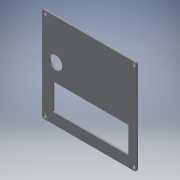
# Autodesk Inventor part: covor
Saved by Autodesk Inventor 2019 (Build 230136000, 136)
## iProperties
Created: 2021-10-12
Part Number: covor
Material: Generic
Document SubType Name: Modeling
Designer: Pulag
Density: 1 g/cm^3
Appearance: Default
Author: Pulag
Autodesk Inventor part; units mm, degrees
ref_plane "YZ Plane" through (0, 0, 0) normal (1, 0, 0) x (0, 1, 0)
ref_plane "XZ Plane" through (0, 0, 0) normal (0, 1, 0) x (-1, 0, 0)
ref_plane "XY Plane" through (0, 0, 0) normal (0, 0, 1) x (1, 0, 0)
sketch "Sketch1" plane through (0, 0, 0) normal (0, 0, 1) x (1, 0, 0)
  arc A0 (-45, -43.5) -> (-43.5, -45) centre (-43.5, -43.5) ccw projected
  line L0 (-43.5, -45) -> (43.5, -45) projected
  arc A1 (43.5, -45) -> (45, -43.5) centre (43.5, -43.5) ccw projected
  line L1 (45, -43.5) -> (45, 4.25) projected
  line L2 (45, 4.25) -> (42.25, 4.25) projected
  line L3 (42.25, 4.25) -> (42.25, -40.75) projected
  arc A2 (40.75, -42.25) -> (42.25, -40.75) centre (42.25, -42.25) ccw projected
  line L4 (40.75, -42.25) -> (-40.75, -42.25) projected
  arc A3 (-42.25, -40.75) -> (-40.75, -42.25) centre (-42.25, -42.25) ccw projected
  line L5 (-42.25, -40.75) -> (-42.25, 40.75) projected
  arc A4 (-40.75, 42.25) -> (-42.25, 40.75) centre (-42.25, 42.25) ccw projected
  line L6 (-40.75, 42.25) -> (-5, 42.25) projected
  line L7 (-5, 42.25) -> (-5, 45) projected
  line L8 (-5, 45) -> (-43.5, 45) projected
  arc A5 (-43.5, 45) -> (-45, 43.5) centre (-43.5, 43.5) ccw projected
  line L9 (-45, 43.5) -> (-45, -43.5) projected
  line L10 (-45, 45) -> (45, 45)
  line L11 (45, 45) -> (45, -45)
  line L12 (45, -45) -> (-45, -45)
  line L13 (-45, -45) -> (-45, 45)
  line L14 (-45, 45) -> (45, -45) construction
  line L15 (45, 45) -> (-45, -45) construction
  line L16 (37.25, -9.75) -> (-34.75, -9.75)
  line L17 (-34.75, -9.75) -> (-34.75, -34.75)
  line L18 (-34.75, -34.75) -> (37.25, -34.75)
  line L19 (37.25, -34.75) -> (37.25, -9.75)
  circle A6 centre (-32, 7) radius 6.25
  point P0 (0, 0)
  dimension "d9" = 1.5
  dimension "d0" = 90
  dimension "d1" = 90
  dimension "d2" = 72
  dimension "d3" = 25
  dimension "d4" = 7.5
  dimension "d5" = 5
  dimension "d6" = 12.5
  dimension "d19" = 38
  dimension "d20" = 13
  constraints: 20 end point, 4 parallel, 2 horizontal, 2 midpoint, 2 perpendicular, 1 centre point
  measures "d0" distance of L10.end L11.end
  measures "d1" distance between parallel lines of L9 L11
  measures "d2" distance of L18.end L17.end
  measures "d3" distance of L17.end L16.end
  measures "d4" distance between parallel lines of L4 L18
  measures "d5" distance between parallel lines of L3 L19
  measures "d6" diameter of A6
  measures "d19" distance from line of L8 A6.centre
  measures "d20" distance from line of L9 A6.centre
extrude "Extrusion1" add sketch "Sketch1" along normal blind 1.5
fillet "Fillet1" radius 2 4 edges at (45, -45, 0.75) (-45, -45, 0.75) (-45, 45, 0.75) (45, 45, 0.75)
sketch "Sketch2" plane through (0, 0, 1.5) normal (0, 0, 1) x (1, 0, 0)
  arc A0 (40.75, -42.25) -> (42.25, -40.75) centre (42.25, -42.25) ccw projected
  arc A1 (-42.25, -40.75) -> (-40.75, -42.25) centre (-42.25, -42.25) ccw projected
  arc A2 (-40.75, 42.25) -> (-42.25, 40.75) centre (-42.25, 42.25) ccw projected
  arc A3 (42.25, 40.75) -> (40.75, 42.25) centre (42.25, 42.25) ccw projected
  circle A4 centre (42.25, 42.25) radius 1.65
  circle A5 centre (-42.25, 42.25) radius 1.65
  circle A6 centre (-42.25, -42.25) radius 1.65
  circle A7 centre (42.25, -42.25) radius 1.65
  point P0 (0, 0)
  dimension "d12" = 3.3
  dimension "d13" = 3.3
  dimension "d14" = 3.3
  dimension "d15" = 3.3
  constraints: 4 centre point, 4 coincident
  measures "d12" diameter of A4
  measures "d13" diameter of A5
  measures "d14" diameter of A6
  measures "d15" diameter of A7
extrude "Extrusion2" cut sketch "Sketch2" against normal blind 3
body "Solid1"
